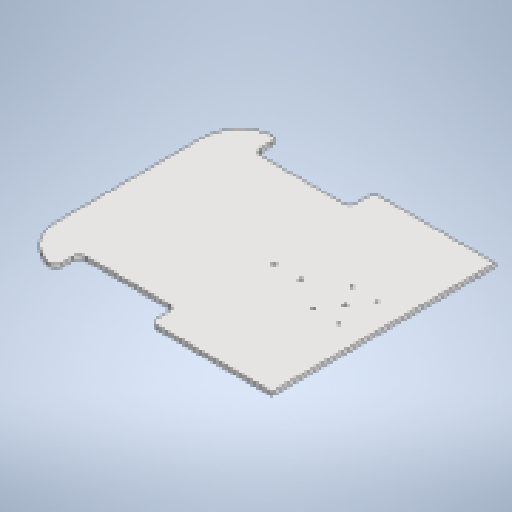
# Autodesk Inventor part: Base_Superior
Saved by Autodesk Inventor 2024 (Build 280153000, 153)
## iProperties
Created: 2025-05-14
Part Number: Base_Superior
Material: Genérico
Document SubType Name: Modeling
Designer: mario
Density: 1 g/cm^3
Appearance: Valor por defecto
Author: mario
Autodesk Inventor part; units mm, degrees
ref_plane "YZ Plane" through (0, 0, 0) normal (1, 0, 0) x (0, 1, 0)
ref_plane "XZ Plane" through (0, 0, 0) normal (0, 1, 0) x (-1, 0, 0)
ref_plane "XY Plane" through (0, 0, 0) normal (0, 0, 1) x (1, 0, 0)
sketch "Boceto1" plane through (0, 0, 0) normal (0, 1, 0) x (-1, 0, 0)
  line L0 (-100, 87.5) -> (100, 87.5)
  line L1 (100, 87.5) -> (100, -87.5)
  line L2 (100, -87.5) -> (-100, -87.5)
  line L3 (-100, -87.5) -> (-100, 87.5)
  line L4 (-100, 87.5) -> (100, -87.5) construction
  line L5 (100, 87.5) -> (-100, -87.5) construction
  point P0 (0, 0)
  dimension "d0" = 200
  dimension "d1" = 175
  constraints: 12 end point, 2 midpoint, 2 parallel, 1 horizontal, 1 perpendicular
  measures "d0" distance of L1.end L2.end
  measures "d1" distance of L0.end L1.end
extrude "Extrusión1" add sketch "Boceto1" along normal blind 3
fillet "Empalme1" radius 30 2 edges at (-100, 1.5, 87.5) (-100, 1.5, -87.5)
sketch "Boceto2" plane through (0, 3, 0) normal (0, 1, 0) x (1, 0, 0)
  line L0 (100, 87.5) -> (-70, 87.5) projected
  line L1 (-70, 87.5) -> (5, 87.5)
  line L2 (5, 87.5) -> (5, 68.5)
  line L3 (5, 68.5) -> (-70, 68.5)
  line L4 (-70, 68.5) -> (-70, 87.5)
  point P0 (0, 0)
  dimension "d5" = 75
  dimension "d6" = 19
  constraints: 8 end point, 2 parallel, 1 perpendicular, 1 point on line
  measures "d5" distance of L2.end L3.end
  measures "d6" distance of L1.end L2.end
extrude "Extrusión2" cut sketch "Boceto2" against normal blind 3
mirror "Simetría1" about plane through (0, 0, 0) normal (0, 0, 1) of "Extrusión2"
fillet "Empalme3" radius 5 8 edges at (-70, 1.5, -87.5) (-70, 1.5, -68.5) (5, 1.5, -87.5) (5, 1.5, -68.5) (5, 1.5, 87.5) (5, 1.5, 68.5) (-70, 1.5, 87.5) (-70, 1.5, 68.5)
sketch "Boceto3" plane through (0, 3, 0) normal (0, 1, 0) x (1, 0, 0)
  line L0 (-100, 57.5) -> (-100, -57.5) construction
  line L1 (-100, 0) -> (100, 0) construction
  line L2 (100, -87.5) -> (100, 87.5) construction
  point P0 (0, 0)
  point P1 (80, 15)
  point P2 (60, 15)
  point P3 (80, -15)
  point P4 (60, -15)
  dimension "d11" = 20
  dimension "d12" = 30
  dimension "d13" = 15
  dimension "d14" = 20
  constraints: 2 end point, 2 midpoint, 2 symmetric about line, 1 horizontal
  measures "d11" distance of point (60, 15) point (80, 15)
  measures "d12" distance of point (80, -15) point (80, 15)
  measures "d13" distance from line of L1 point (60, 15)
  measures "d14" distance from line of L2 point (80, 15)
hole "Agujero1" at (80, 3, -15) at (60, 3, -15) at (60, 3, 15) at (80, 3, 15) direction (0, -1, 0) diameter 3 end through all
sketch "Boceto5" plane through (0, 3, 0) normal (0, 1, 0) x (1, 0, 0)
  circle A0 centre (60, -15) radius 1.5 construction
  point P0 (0, 0)
  point P1 (70, 0)
  dimension "d22" = 15
  dimension "d23" = 10
  measures "d22" vertical distance of A0.centre point (70, 0)
  measures "d23" horizontal distance of A0.centre point (70, 0)
hole "Agujero2" at (70, 3, 0) direction (0, -1, 0) diameter 2.5 end through all
sketch "Boceto6" plane through (0, 3, 0) normal (0, 1, 0) x (1, 0, 0)
  line L0 (100, -87.5) -> (100, 87.5) construction
  line L1 (100, 0) -> (-100, 0) construction
  line L2 (-100, 57.5) -> (-100, -57.5) construction
  point P0 (0, 0)
  point P1 (35, 0)
  point P2 (14, 0)
  dimension "d31" = 21
  dimension "d32" = 65
  constraints: 2 end point, 2 midpoint, 2 point on line
  measures "d31" distance of point (35, 0) point (14, 0)
  measures "d32" distance from line of L0 point (35, 0)
hole "Agujero3" at (35, 3, 0) at (14, 3, 0) direction (0, -1, 0) diameter 3 end through all
sketch "Boceto7" plane through (0, 3, 0) normal (0, 1, 0) x (1, 0, 0)
  line L0 (-90, 66.5) -> (-90, -66.5) construction
  line L1 (15, -77.5) -> (90, -77.5) construction
  line L2 (15, 77.5) -> (90, 77.5) construction
  line L3 (10, -87.5) -> (100, -87.5) construction
  line L4 (100, -87.5) -> (100, 87.5) construction
  line L5 (5, -73.5) -> (5, -82.5) construction
  line L6 (100, 87.5) -> (10, 87.5) construction
  line L7 (-100, 57.5) -> (-100, -57.5) construction
  line L8 (-65, -68.5) -> (0, -68.5) construction
  point P0 (0, 0)
  point P1 (-90, 0)
  dimension "d40" = 10
  dimension "d41" = 10
  dimension "d42" = 10
  dimension "d43" = 10
  dimension "d44" = 10
  dimension "d45" = 2
  constraints: 6 end point, 2 horizontal, 1 horizontal alignment, 1 midpoint, 1 parallel, 1 vertical, 1 vertical alignment
  measures "d40" distance from line of L3 L1.start
  measures "d41" distance from line of L4 L1.end
  measures "d42" distance from line of L5 L1.start
  measures "d43" distance between parallel lines of L6 L2
  measures "d44" distance between parallel lines of L7 L0
  measures "d45" distance from line of L8 L0.end
hole "Agujero4" at (-90, 3, 66.5) at (-90, 3, -66.5) at (90, 3, 77.5) at (90, 3, -77.5) at (15, 3, 77.5) at (15, 3, -77.5) direction (0, -1, 0) diameter 3 depth 8 tip angle 118
sketch "Boceto8" plane through (0, 3, 0) normal (0, 1, 0) x (1, 0, 0)
  line L0 (-100, 57.5) -> (-100, -57.5) projected
  point P0 (0, 0)
  point P1 (-70, 25)
  point P2 (-18.1608, 8.6361)
  point P3 (-18.1608, -18.8802)
  point P4 (-70, -24.5)
  point P5 (-100, 0)
  dimension "d53" = 49.5
  dimension "d54" = 51.8392
  dimension "d55" = 16.3639
  dimension "d56" = 27.5163
  dimension "d57" = 30
  dimension "d58" = 25
  constraints: 2 vertical alignment, 1 midpoint
  measures "d53" distance of point (-70, -24.5) point (-70, 25)
  measures "d54" horizontal distance of point (-18.161, 8.636) point (-70, 25)
  measures "d55" vertical distance of point (-70, 25) point (-18.161, 8.636)
  measures "d56" distance of point (-18.161, -18.88) point (-18.161, 8.636)
  measures "d57" distance from line of L0 point (-70, 25)
  measures "d58" vertical distance of point (-100, 0) point (-70, 25)
hole "Agujero5" at (-70, 3, -25) at (-18.1608, 3, -8.6361) at (-18.1608, 3, 18.8802) at (-70, 3, 24.5) direction (0, -1, 0) diameter 3 end through all
sketch "Boceto9" plane through (0, 3, 0) normal (0, 1, 0) x (1, 0, 0)
  line L0 (-17, 40) -> (-67, 40)
  line L1 (-67, 40) -> (-67, 35)
  line L2 (-67, 35) -> (-17, 35)
  line L3 (-17, 35) -> (-17, 40)
  line L4 (-100, 57.5) -> (-100, -57.5) projected
  point P0 (0, 0)
  point P1 (-100, 0)
  dimension "d66" = 5
  dimension "d67" = 33
  dimension "d68" = 50
  dimension "d69" = 35
  constraints: 8 end point, 2 parallel, 1 horizontal, 1 midpoint, 1 perpendicular
  measures "d66" distance of L1.end L0.end
  measures "d67" distance between parallel lines of L4 L1
  measures "d68" distance of L0.start L0.end
  measures "d69" distance from line of point (-100, 0) L2
extrude "Extrusión3" cut sketch "Boceto9" against normal through all
sketch "Boceto10" plane through (0, 3, 0) normal (0, 1, 0) x (1, 0, 0)
  line L0 (-17, -33) -> (-55, -33)
  line L1 (-55, -33) -> (-55, -38)
  line L2 (-55, -38) -> (-17, -38)
  line L3 (-17, -38) -> (-17, -33)
  line L4 (-17, 35) -> (-67, 35) construction
  point P0 (0, 0)
  dimension "d72" = 5
  dimension "d73" = 68
  dimension "d74" = 38
  constraints: 8 end point, 2 parallel, 1 horizontal, 1 perpendicular, 1 vertical alignment
  measures "d72" distance of L1.end L0.end
  measures "d73" distance between parallel lines of L4 L0
  measures "d74" distance of L1.end L2.end
extrude "Extrusión4" cut sketch "Boceto10" against normal through all
sketch "Boceto11" plane through (0, 3, 0) normal (0, 1, 0) x (1, 0, 0)
  line L0 (-100, 57.5) -> (-100, -57.5) projected
  line L1 (-65, -68.5) -> (0, -68.5) projected
  point P0 (0, 0)
  point P1 (-65, -48.5)
  dimension "d77" = 35
  dimension "d78" = 20
  measures "d77" distance from line of L0 point (-65, -48.5)
  measures "d78" distance from line of L1 point (-65, -48.5)
hole "Agujero6" at (-65, 3, 48.5) direction (0, -1, 0) diameter 4 end through all
